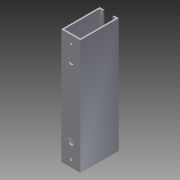
# Autodesk Inventor part: 07
Saved by Autodesk Inventor 2013 (Build 170138000, 138)
## iProperties
Created: 2014-02-11
Material: アルミニウム 6061
Document SubType Name: Modeling
Designer: andou
Density: 2.71 g/cm^3
Mass: 43.0344 g
Surface Area: 168.079 cm^2
Volume: 15.8798 cm^3
Part Number: 07
Author: andou
Title: Long_Serial_Case
Autodesk Inventor part; units mm, degrees
ref_plane "YZ Plane" through (0, 0, 0) normal (1, 0, 0) x (0, 1, 0)
ref_plane "XZ Plane" through (0, 0, 0) normal (0, 1, 0) x (-1, 0, 0)
ref_plane "XY Plane" through (0, 0, 0) normal (0, 0, 1) x (1, 0, 0)
sketch "スケッチ1" plane through (0, 0, 0) normal (0, 0, 1) x (1, 0, 0)
  line L0 (-12.5, 25) -> (12.5, 25)
  line L1 (12.5, 25) -> (12.5, -25)
  line L2 (12.5, -25) -> (-12.5, -25)
  line L3 (-12.5, -25) -> (-12.5, 25)
  line L4 (-10.5, 23) -> (10.5, 23)
  line L5 (10.5, 23) -> (10.5, -23)
  line L6 (10.5, -23) -> (-10.5, -23)
  line L7 (-10.5, -23) -> (-10.5, 23)
  point P0 (0, 0)
  dimension "d0" = 25
  dimension "d1" = 50
  dimension "d2" = 46
  dimension "d3" = 21
  dimension "d4" = 25
  dimension "d5" = 23
  dimension "d6" = 10.5
  dimension "d7" = 12.5
  constraints: 16 end point, 4 parallel, 2 horizontal, 2 perpendicular
  measures "d0" distance of L0.start L0.end
  measures "d1" distance of L2.end L0.start
  measures "d2" distance of L6.end L4.start
  measures "d3" distance of L4.start L4.end
  measures "d4" distance from line of L0 point (0, 0)
  measures "d5" distance from line of point (0, 0) L6
  measures "d6" distance from line of point (0, 0) L7
  measures "d7" distance from line of point (0, 0) L1
extrude "押し出し1" add sketch "スケッチ1" along normal blind 150
sketch "スケッチ2" plane through (-12.5, 25, 0) normal (0, 1, 0) x (1, 0, 0)
  line L0 (0, 0) -> (25, 0) projected
  line L1 (0, 0) -> (0, -150) projected
  arc A0 (6, -32.5) -> (19, -32.5) centre (12.5, -32.5) ccw
  line L2 (6, -32.5) -> (6, 0)
  line L3 (19, -32.5) -> (19, 0)
  point P0 (12.5, 0)
  dimension "d10" = 13
  dimension "d11" = 32.5
  dimension "d12" = 12.5
  constraints: 4 end point, 2 perpendicular, 2 point on circle, 2 point on line, 2 tangent, 1 centre point
  measures "d10" diameter of A0
  measures "d11" distance from line of L0 A0.centre
  measures "d12" distance from line of L1 A0.centre
extrude "押し出し2" cut sketch "スケッチ2" against normal blind 2
sketch "スケッチ3" plane through (-12.5, 25, 150) normal (0, 1, 0) x (1, 0, 0)
  arc A0 (6, 117.5) -> (19, 117.5) centre (12.5, 117.5) ccw projected
  circle A1 centre (4.5, 111) radius 1
  circle A2 centre (4.5, 147) radius 1
  circle A3 centre (20.5, 147) radius 1
  circle A4 centre (20.5, 111) radius 1
  point P0 (12.5, 150)
  dimension "d15" = 6.5
  dimension "d16" = 6.5
  dimension "d17" = 2
  dimension "d18" = 8
  dimension "d19" = 8
  dimension "d20" = 8
  dimension "d21" = 8
  dimension "d22" = 29.5
  dimension "d23" = 29.5
  constraints: 4 centre point, 3 equal radius
  measures "d15" vertical distance of A0.centre A1.centre
  measures "d16" vertical distance of A0.centre A4.centre
  measures "d17" diameter of A1
  measures "d18" horizontal distance of A0.centre A2.centre
  measures "d19" horizontal distance of A0.centre A3.centre
  measures "d20" horizontal distance of A0.centre A4.centre
  measures "d21" horizontal distance of A0.centre A1.centre
  measures "d22" vertical distance of A3.centre A0.centre
  measures "d23" vertical distance of A2.centre A0.centre
hole "穴1" at (-8, 25, 3) at (8, 25, 3) at (8, 25, 39) at (-8, 25, 39) direction (0, -1, 0) diameter 2 depth 2 tip angle 118 counterbore diameter 4 counterbore depth 0.5
sketch "スケッチ4" plane through (-12.5, -25, 0) normal (0, -1, 0) x (1, 0, 0)
  line L0 (25, 0) -> (0, 0) projected
  line L1 (25, 0) -> (25, 150) projected
  circle A0 centre (12.5, 9.5) radius 2
  point P0 (12.5, 0)
  dimension "d31" = 4
  dimension "d32" = 12.5
  dimension "d33" = 9.5
  constraints: 1 centre point
  measures "d31" diameter of A0
  measures "d32" distance from line of A0.centre L1
  measures "d33" distance from line of L0 A0.centre
hole "穴2" at (0, -25, 9.5) direction (0, 1, 0) diameter 4 end through all
sketch "スケッチ7" plane through (-12.5, -25, 0) normal (0, -1, 0) x (1, 0, 0)
  line L0 (25, 0) -> (25, 150) projected
  circle A0 centre (12.5, 29) radius 4
  line L1 (25, 0) -> (0, 0) projected
  point P0 (12.5, 0)
  dimension "d79" = 8
  dimension "d80" = 12.5
  dimension "d88" = 29
  constraints: 1 centre point
  measures "d79" diameter of A0
  measures "d80" distance from line of L0 A0.centre
  measures "d88" distance from line of A0.centre L1
hole "穴5" at (0, -25, 29) direction (0, 1, 0) diameter 8 end through all
sketch "スケッチ9" plane through (-12.5, 25, 150) normal (0, 1, 0) x (1, 0, 0)
  line L0 (0, 150) -> (0, 0) projected
  line L1 (0, 0) -> (25, 0) projected
  line L2 (6, 0) -> (19, 0)
  line L3 (19, 0) -> (19, 32.5)
  line L4 (6, 32.5) -> (6, 0)
  arc A0 (19, 32.5) -> (6, 32.5) centre (12.5, 32.5) ccw
  point P0 (12.5, 150)
  dimension "d92" = 13
  dimension "d93" = 12.5
  dimension "d95" = 32.5
  dimension "d96" = 6.5
  dimension "d97" = 6.5
  constraints: 6 end point, 2 point on circle, 1 centre point, 1 horizontal, 1 parallel, 1 perpendicular, 1 point on line
  measures "d92" distance between parallel lines of L3 L4
  measures "d93" distance from line of L0 A0.centre
  measures "d95" distance from line of A0.centre L2
  measures "d96" radius of A0
  measures "d97" distance from line of A0.centre L3
extrude "押し出し4" cut sketch "スケッチ9" against normal blind 2
sketch "スケッチ10" plane through (12.5, 25, 150) normal (0, 1, 0) x (1, 0, 0)
  arc A0 (-6, 32.5) -> (-19, 32.5) centre (-12.5, 32.5) ccw projected
  circle A1 centre (-20.5, 39) radius 1
  circle A2 centre (-20.5, 3) radius 1
  circle A3 centre (-4.5, 3) radius 1
  circle A4 centre (-4.5, 39) radius 1
  point P0 (-12.5, 150)
  dimension "d100" = 2
  dimension "d102" = 16
  dimension "d103" = 16
  dimension "d106" = 8
  dimension "d110" = 8
  dimension "d138" = 6.5
  dimension "d139" = 6.5
  dimension "d140" = 29.5
  dimension "d141" = 29.5
  constraints: 4 centre point, 3 equal radius
  measures "d100" diameter of A4
  measures "d102" distance of A4.centre A1.centre
  measures "d103" distance of A3.centre A2.centre
  measures "d106" horizontal distance of A0.centre A3.centre
  measures "d110" horizontal distance of A0.centre A1.centre
  measures "d138" vertical distance of A1.centre A0.centre
  measures "d139" vertical distance of A4.centre A0.centre
  measures "d140" vertical distance of A0.centre A2.centre
  measures "d141" vertical distance of A0.centre A3.centre
hole "穴6" at (8, 25, 147) at (-8, 25, 147) at (-8, 25, 111) at (8, 25, 111) direction (0, -1, 0) diameter 2 depth 2 tip angle 118 counterbore diameter 4 counterbore depth 0.5
sketch "スケッチ11" plane through (-12.5, -25, 0) normal (0, -1, 0) x (1, 0, 0)
  line L0 (25, 150) -> (0, 150) projected
  line L1 (25, 0) -> (25, 150) projected
  circle A0 centre (12.5, 140.5) radius 2
  point P0 (12.5, 0)
  dimension "d118" = 9.5
  dimension "d119" = 4
  dimension "d120" = 12.5
  constraints: 1 centre point
  measures "d118" distance from line of L0 A0.centre
  measures "d119" diameter of A0
  measures "d120" distance from line of L1 A0.centre
hole "穴7" at (0, -25, 140.5) direction (0, 1, 0) diameter 4 depth 2 tip angle 118
sketch "スケッチ12" plane through (-12.5, -25, 0) normal (0, -1, 0) x (1, 0, 0)
  line L0 (25, 150) -> (0, 150) projected
  line L1 (25, 0) -> (25, 150) projected
  circle A0 centre (12.5, 120) radius 4
  point P0 (12.5, 0)
  dimension "d128" = 30
  dimension "d129" = 8
  dimension "d130" = 12.5
  constraints: 1 centre point
  measures "d128" distance from line of L0 A0.centre
  measures "d129" diameter of A0
  measures "d130" distance from line of L1 A0.centre
hole "穴8" at (0, -25, 120) direction (0, 1, 0) diameter 8 depth 2 tip angle 118
